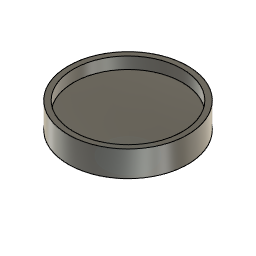
INJECTOR PLATE (FIRST DESIGN RAW) v1 (Autodesk Fusion 360 design; units mm, degrees)
Autodesk Fusion 360 part; units mm, degrees
sketch "Sketch1" plane through (0, 0, 0) normal (0, 0, 1) x (1, 0, 0)
  circle A0 centre (0, 0) radius 50
  constraint coincident A0.centre origin
extrude "Extrude1" add sketch "Sketch1" along normal blind 20
ref_plane "WorkPlane1" through (0, 0, 10) normal (0, 0, 1) x (1, 0, 0)
sketch "Sketch2" plane through (0, 0, 10) normal (0, 0, 1) x (1, 0, 0)
  circle A0 centre (0, 0) radius 47.5
  constraint coincident A0.centre origin
extrude "Extrude2" cut sketch "Sketch2" along normal blind 10
sketch "Sketch3" plane through (0, 0, 0) normal (0, 0, 1) x (1, 0, 0)
  circle A0 centre (0, 0) radius 20
  constraint coincident A0.centre origin
extrude "Extrude3" add sketch "Sketch3" against normal blind 20
sketch "Sketch4" plane through (0, 0, -20) normal (0, 0, -1) x (1, 0, 0)
  circle A0 centre (0, 0) radius 20
shell "Shell1" thickness 1 outward yes removed faces 1 at (6.3705, -1.965, -20)
